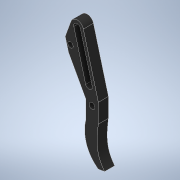
# Autodesk Inventor part: Abzug
Saved by Autodesk Inventor 2021 (Build 250183000, 183)
## iProperties
Created: 2021-03-08
Part Number: Abzug
Material: Generic
Document SubType Name: Modeling
Designer: Lukas
Density: 1 g/cm^3
Appearance: Default
Author: Lukas
Autodesk Inventor part; units mm, degrees
ref_plane "YZ Plane" through (0, 0, 0) normal (1, 0, 0) x (0, 1, 0)
ref_plane "XZ Plane" through (0, 0, 0) normal (0, 1, 0) x (-1, 0, 0)
ref_plane "XY Plane" through (0, 0, 0) normal (0, 0, 1) x (1, 0, 0)
sketch "Sketch1" plane through (0, 0, 0) normal (0, 0, 1) x (1, 0, 0)
  line L0 (-3, -1.5) -> (-3, -10.5)
  line L1 (3, 0) -> (3, -9)
  line L2 (-3, -10.5) -> (-4, -14.5) construction
  line L3 (-4, -14.5) -> (-4, -22.5) construction
  line L4 (-4, -22.5) -> (3, -27.5) construction
  spline S0 degree 3 poles (-3, -10.5) (-4, -14.5) (-4, -22.5) (3, -27.5) knots 1 1 1 1 2 2 2 2
  line L5 (3, -27.5) -> (6, -27)
  line L6 (6, -27) -> (2, -22) construction
  line L7 (2, -22) -> (2, -17) construction
  line L8 (2, -17) -> (3, -9) construction
  spline S1 degree 3 poles (6, -27) (2, -22) (2, -17) (3, -9) knots 1 1 1 1 2 2 2 2
  line L9 (-3, -1.5) -> (-10.0906, 24.9625)
  arc A0 (-4.1175, 26.563) -> (-10.0906, 24.9625) centre (-7.1041, 25.7627) ccw
  line L10 (-4.1175, 26.563) -> (3, 0)
  line L11 (-7.1041, 25.7627) -> (-1.4806, 4.7757) construction
  line L12 (-8.6495, 25.3486) -> (-3.0261, 4.3616)
  line L13 (0.0649, 5.1899) -> (-5.5586, 26.1768)
  arc A1 (-5.5586, 26.1768) -> (-8.6495, 25.3486) centre (-7.1041, 25.7627) ccw
  arc A2 (-3.0261, 4.3616) -> (0.0649, 5.1899) centre (-1.4806, 4.7757) ccw
  circle A3 centre (0, -3) radius 1.4
  line L14 (-10.0138, 26.8082) -> (-12.7133, 19.2956)
  line L15 (-12.7133, 19.2956) -> (-11.1603, 13.5)
  line L16 (-11.1603, 13.5) -> (-3, -1.5)
  circle A4 centre (-10.2347, 17) radius 1.25
  point P0 (0, 0)
  point P1 (-4.2923, 15.2692)
  dimension "d8" = 1
  dimension "d9" = 3
  dimension "d10" = 3
  dimension "d11" = 18
  dimension "d12" = 8
  dimension "d13" = 5
  dimension "d15" = 0.5
  dimension "d17" = 1
  dimension "d18" = 4
  dimension "d19" = 8
  dimension "d25" = 6
  dimension "d26" = 3
  dimension "d27" = 9
  dimension "d61" = 3.2
  dimension "d62" = 27.5
  dimension "d63" = 5
  dimension "d64" = 2.8
  dimension "d65" = 3
  dimension "d68" = 6
  dimension "d69" = 1.8
  dimension "d70" = 2.5
  dimension "d72" = 4
  dimension "d73" = 15
  dimension "d74" = 15
  dimension "d75" = 3.5
  dimension "d76" = 1.5
  constraints: 24 end point, 7 point on circle, 7 tangent, 5 centre point, 5 parallel, 3 vertical, 3 vertical alignment, 1 horizontal alignment, 1 midpoint, 6 other
  measures "d8" distance from line of L1 L7.end
  measures "d9" distance from line of L1 L5.end
  measures "d10" horizontal distance of L5.end L4.end
  measures "d11" vertical distance of L1.end L5.end
  measures "d12" vertical distance of L1.end L7.end
  measures "d13" distance of L7.end L6.end
  measures "d15" vertical distance of L5.end L4.end
  measures "d17" distance from line of L0 L2.end
  measures "d18" vertical distance of L0.end L2.end
  measures "d19" distance of L3.end L2.end
  measures "d25" distance between parallel lines of L0 L1
  measures "d26" distance from line of point (0, 0) L1
  measures "d27" distance of L0.start L0.end
  measures "d61" distance between parallel lines of L13 L12
  measures "d62" distance of L10.start L1.start
  measures "d63" distance of point (0, 0) L11.end
  measures "d64" diameter of A3
  measures "d65" distance of point (0, 0) A3.centre
  measures "d68" distance of L14.end L15.end
  measures "d69" distance from line of L15 A4.centre
  measures "d70" diameter of A4
  measures "d72" distance between parallel lines of L9 L15
  measures "d73" angle of L1 L10
  measures "d74" vertical distance of L15.end L0.start
  measures "d75" vertical distance of L15.end A4.centre
  measures "d76" vertical distance of point (0, 0) L0.start
extrude "Extrusion1" add sketch "Sketch1" along normal mid plane 4.8
equation "\"d26\" = 0.5 * d25"
body "Solid1"
